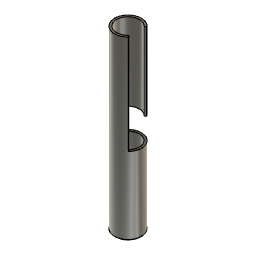
basemarcador2 v15 (Autodesk Fusion 360 design; units mm, degrees)
Autodesk Fusion 360 part; units mm, degrees
note: some values were not read from the file. Set by a fixed rule: which face or edge a step refers to.
sketch "Boceto2" plane through (0, 0, 0) normal (0, 0, 1) x (1, 0, 0)
  circle A0 centre (0, 0) radius 11.25
  circle A1 centre (0, 0) radius 9.5
  dimension "d14" = 22.5
  dimension "d15" = 19
  constraint coincident A0.centre A1.centre
  measures "d14" diameter of A0
  measures "d15" diameter of A1
extrude "Extruir2" add sketch "Boceto2" along normal blind 144
sketch "Boceto3" plane through (0, 0, 0) normal (0, 0, 1) x (1, 0, 0)
  circle A0 centre (0, 0) radius 11.25
  dimension "d16" = 22.5
  constraint coincident A0.centre origin
  measures "d16" diameter of A0
extrude "Extruir3" add sketch "Boceto3" against normal blind 3
sketch "Boceto5" plane through (0, 0, 0) normal (1, 0, 0) x (0, 1, 0)
sketch "Boceto6" plane through (0, 0, 0) normal (1, 0, 0) x (0, 1, 0)
  line L0 (0, 0) -> (0, 129.72)
  line L1 (0, 129.72) -> (-8.75, 129.72)
  circle A0 centre (-8.75, 129.72) radius 1
  circle A1 centre (8.75, 129.72) radius 1
  dimension "d28" = 129.72
  dimension "d29" = 8.75
  dimension "d30" = 2
  constraint coincident L0.start origin
  constraint vertical L0
  constraint perpendicular L0 L1
  constraint coincident L1.end A0.centre
  constraint symmetric L0 A0 A1
  measures "d28" distance of L0.start L0.end
  measures "d29" distance of L0.end L1.end
  measures "d30" diameter of A0
sketch "Boceto7" plane through (0, 0, 0) normal (1, 0, 0) x (0, 1, 0)
  line L0 (0, 0) -> (0, 61.5)
  line L1 (0, 61.5) -> (27.6846, 61.5)
  line L2 (27.6846, 61.5) -> (0, 61.5)
  line L3 (0, 61.5) -> (0, 79.5)
  line L4 (0, 79.5) -> (27.6846, 79.5)
  line L5 (27.6846, 79.5) -> (27.6846, 61.5)
  dimension "d33" = 61.5
  dimension "d34" = 27.6846
  dimension "d35" = 18
  constraint coincident L0.start origin
  constraint vertical L0
  constraint perpendicular L0 L1
  constraint horizontal L2
  constraint vertical L3
  constraint horizontal L4
  constraint vertical L5
  measures "d33" distance of L0.start L0.end
  measures "d34" distance of L0.end L1.end
  measures "d35" distance of L1.end L4.end
emboss "Repujado1" depth -2 profiles "Boceto7" section 1 onto face at (11.236, -0.5608, 96)
fillet "Empalme4" radius 1 1 edges at (-10.4887, 4.0682, -3)
ref_plane "PlanoDeObra1" through (11.25, 0, 101.1607) normal (1, 0, 0) x (0, -1, 0)
sketch "Boceto8" plane through (11.25, 0, 0) normal (1, 0, 0) x (0, 1, 0)
  line L0 (0, 0) -> (0, 70.5)
  line L1 (0, 70.5) -> (9, 70.5)
  line L2 (9, 70.5) -> (9, 144)
  line L3 (9, 144) -> (0, 144)
  line L4 (0, 70.5) -> (-9, 70.5)
  line L5 (-9, 70.5) -> (-9, 144)
  line L6 (-9, 144) -> (0, 144)
  line L7 (9, 70.5) -> (9, 61.5)
  line L8 (9, 61.5) -> (-9, 61.5)
  line L9 (-9, 70.5) -> (-9, 61.5)
  dimension "d51" = 70.5
  dimension "d52" = 9
  dimension "d53" = 73.5
  dimension "d54" = 9
  dimension "d55" = 9
  dimension "d56" = 18
  constraint coincident L0.start origin
  constraint vertical L0
  constraint perpendicular L0 L1
  constraint perpendicular L1 L2
  constraint perpendicular L2 L3
  constraint symmetric L1.start L0 L4.start
  constraint symmetric L0 L1.end L4.end
  constraint symmetric L0 L2.end L5.end
  constraint symmetric L0 L3.end L6.end
  constraint perpendicular L1 L7
  constraint perpendicular L0 L8
  measures "d51" distance of L0.start L0.end
  measures "d52" distance of L0.end L1.end
  measures "d53" distance of L1.end L2.end
  measures "d54" distance of L2.end L3.end
  measures "d55" distance of L1.end L7.end
  measures "d56" distance of L7.end L8.end
extrude "Extruir5" cut sketch "Boceto8" against normal blind 3
fillet "Empalme5" radius 1 2 edges at (8.25, -4.7104, 102.75) (8.25, -7.6485, 102.75)
fillet "Empalme6" radius 1 2 edges at (8.25, 7.6485, 111.75) (8.25, 4.7104, 111.75)
equation "Lm = 120 mm" comment "Largo marcador"
equation "lr = 15 mm" comment "largo resorte"
equation "e1 = 3 mm" comment "espesor"
equation "gm = 15 mm" comment "grosor marcador"
equation "gp = 6 mm" comment "grosor punta"
equation "gb = 15 mm" comment "grosor base"
equation "e2 = 3 mm" comment "espesor 2"
equation "gs = 2 mm" comment "grosor seguro"
equation "Ds = 1.5 mm" comment "distancia seguro"
equation "d12 = ( Lm + lr + ( e1 + 3 mm + 3 mm ) )"
equation "d14 = ( gm + ( e1 / 2 ) ) + e1 + ( e1 )"
equation "d15 = ( gm ) + e1 + 1 mm"
equation "d16 = ( gm + ( e1 / 2 ) ) + e1 + ( e1 )"
equation "d17 = -e1"
equation "d28 = ( Lm + lr + ( e1 + 3 mm ) ) * 0.92"
equation "d30 = gs"
equation "d33 = ( ( Lm + lr + ( e1 + 3 mm ) ) / 2 ) - 9 mm"
equation "d34 = ( ( 3.141516 / 2 ) ) * ( ( ( gm + ( e1 / 2 ) + e1 ) + 1 mm + ( e1 ) ) / 2 ) * 1.5"
equation "x = 18 mm" comment "grosror ajuste"
equation "d51 = ( ( Lm + lr + ( e1 + 3 mm ) ) / 2 )"
equation "d53 = ( ( Lm + lr + ( e1 + 3 mm ) ) / 2 ) + 3 mm"
equation "d57 = -e1"
